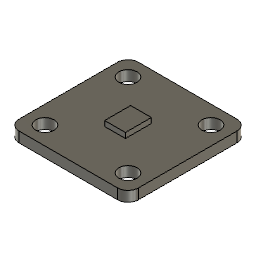
Leg Assembly 2026-01-18 (Autodesk Fusion 360 archive; units mm, degrees)
design "encoderBB"
Autodesk Fusion 360 part; units mm, degrees
sketch "Sketch1" plane through (0, 0, 0) normal (0, 0, 1) x (1, 0, 0)
  line L0 (8, -8) -> (-8, -8)
  line L1 (-8, -8) -> (-8, 8)
  line L2 (-8, 8) -> (8, 8)
  line L3 (8, 8) -> (8, -8)
  line L4 (8, -8) -> (-8, 8) construction
  line L5 (-8, -8) -> (8, 8) construction
  circle A0 centre (-8, 8) radius 1.75
  circle A1 centre (-8, -8) radius 1.75
  circle A2 centre (8, -8) radius 1.75
  circle A3 centre (8, 8) radius 1.75
  line L6 (11.5, -11.5) -> (-11.5, -11.5)
  line L7 (-11.5, -11.5) -> (-11.5, 11.5)
  line L8 (-11.5, 11.5) -> (11.5, 11.5)
  line L9 (11.5, 11.5) -> (11.5, -11.5)
  line L10 (11.5, -11.5) -> (-11.5, 11.5) construction
  line L11 (-11.5, -11.5) -> (11.5, 11.5) construction
  dimension "d1" = 16
  dimension "d2" = 16
  dimension "d3" = 3.5
  dimension "d4" = 3.5
  dimension "d5" = 3.5
  dimension "d6" = 3.5
  dimension "d7" = 23
  dimension "d8" = 23
  constraint horizontal L0
  constraint perpendicular L0 L1
  constraint parallel L0 L2
  constraint parallel L1 L3
  constraint coincident L4 origin
  constraint coincident L5 origin
  constraint coincident L1.end L2.start
  constraint coincident L0.end L1.start
  constraint coincident L0.start L3.end
  constraint coincident L2.end L3.start
  constraint horizontal L6
  constraint perpendicular L6 L7
  constraint parallel L6 L8
  constraint parallel L7 L9
  constraint coincident L10 origin
  constraint coincident L11 origin
  measures "d1" distance of L1.end L2.end
  measures "d2" distance of L0.end L1.end
  measures "d3" diameter of A0
  measures "d4" diameter of A1
  measures "d5" diameter of A2
  measures "d6" diameter of A3
  measures "d7" distance of L7.end L8.end
  measures "d8" distance of L6.end L7.end
extrude "Extrude1" add sketch "Sketch1" along normal blind 2 contours L0 L1 L2 L3 A0 A1 A2 A3 | L6 L7 L8 L9
fillet "Fillet1" radius 2 4 edges at (-11.5, 11.5, 1) (-11.5, -11.5, 1) (11.5, -11.5, 1) (11.5, 11.5, 1)
sketch "Sketch2" plane through (0, 0, 2) normal (0, 0, 1) x (-1, 0, 0)
  arc A0 (-11.5, -9.5) -> (-9.5, -11.5) centre (-9.5, -9.5) ccw
  line L0 (-9.5, -11.5) -> (9.5, -11.5)
  arc A1 (9.5, -11.5) -> (11.5, -9.5) centre (9.5, -9.5) ccw
  line L1 (11.5, -9.5) -> (11.5, 9.5)
  arc A2 (11.5, 9.5) -> (9.5, 11.5) centre (9.5, 9.5) ccw
  line L2 (9.5, 11.5) -> (-9.5, 11.5)
  arc A3 (-9.5, 11.5) -> (-11.5, 9.5) centre (-9.5, 9.5) ccw
  line L3 (-11.5, 9.5) -> (-11.5, -9.5)
  circle A4 centre (-8, -8) radius 1.75
  circle A5 centre (8, 8) radius 1.75
  circle A6 centre (-8, 8) radius 1.75
  circle A7 centre (8, -8) radius 1.75
  line L4 (-2, 2.5) -> (2, 2.5)
  line L5 (2, 2.5) -> (2, -2.5)
  line L6 (2, -2.5) -> (-2, -2.5)
  line L7 (-2, -2.5) -> (-2, 2.5)
  line L8 (-2, 2.5) -> (2, -2.5) construction
  line L9 (2, 2.5) -> (-2, -2.5) construction
  dimension "d13" = 4
  dimension "d14" = 5
  constraint horizontal L4
  constraint perpendicular L4 L5
  constraint parallel L4 L6
  constraint parallel L5 L7
  constraint coincident L8 origin
  constraint coincident L9 origin
  measures "d13" distance of L5.end L6.end
  measures "d14" distance of L4.end L5.end
extrude "Extrude2" add sketch "Sketch2" along normal blind 1 contours L4 L5 L6 L7

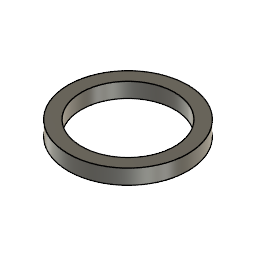
design "25mm id bearing"
Autodesk Fusion 360 part; units mm, degrees
sketch "Sketch1" plane through (0, 0, 0) normal (0, 0, 1) x (1, 0, 0)
  circle A0 centre (0, 0) radius 12.5
  circle A1 centre (0, 0) radius 16
  dimension "d1" = 25
  dimension "d2" = 32
  constraint coincident A0.centre A1.centre
  measures "d1" diameter of A0
  measures "d2" diameter of A1
extrude "Extrude1" add sketch "Sketch1" along normal blind 4

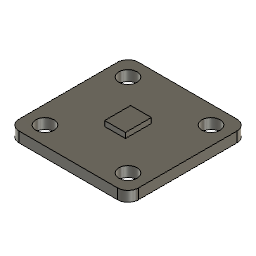
design "encoderBB"
Autodesk Fusion 360 part; units mm, degrees
sketch "Sketch1" plane through (0, 0, 0) normal (0, 0, 1) x (1, 0, 0)
  line L0 (8, -8) -> (-8, -8)
  line L1 (-8, -8) -> (-8, 8)
  line L2 (-8, 8) -> (8, 8)
  line L3 (8, 8) -> (8, -8)
  line L4 (8, -8) -> (-8, 8) construction
  line L5 (-8, -8) -> (8, 8) construction
  circle A0 centre (-8, 8) radius 1.75
  circle A1 centre (-8, -8) radius 1.75
  circle A2 centre (8, -8) radius 1.75
  circle A3 centre (8, 8) radius 1.75
  line L6 (11.5, -11.5) -> (-11.5, -11.5)
  line L7 (-11.5, -11.5) -> (-11.5, 11.5)
  line L8 (-11.5, 11.5) -> (11.5, 11.5)
  line L9 (11.5, 11.5) -> (11.5, -11.5)
  line L10 (11.5, -11.5) -> (-11.5, 11.5) construction
  line L11 (-11.5, -11.5) -> (11.5, 11.5) construction
  dimension "d1" = 16
  dimension "d2" = 16
  dimension "d3" = 3.5
  dimension "d4" = 3.5
  dimension "d5" = 3.5
  dimension "d6" = 3.5
  dimension "d7" = 23
  dimension "d8" = 23
  constraint horizontal L0
  constraint perpendicular L0 L1
  constraint parallel L0 L2
  constraint parallel L1 L3
  constraint coincident L4 origin
  constraint coincident L5 origin
  constraint coincident L1.end L2.start
  constraint coincident L0.end L1.start
  constraint coincident L0.start L3.end
  constraint coincident L2.end L3.start
  constraint horizontal L6
  constraint perpendicular L6 L7
  constraint parallel L6 L8
  constraint parallel L7 L9
  constraint coincident L10 origin
  constraint coincident L11 origin
  measures "d1" distance of L1.end L2.end
  measures "d2" distance of L0.end L1.end
  measures "d3" diameter of A0
  measures "d4" diameter of A1
  measures "d5" diameter of A2
  measures "d6" diameter of A3
  measures "d7" distance of L7.end L8.end
  measures "d8" distance of L6.end L7.end
extrude "Extrude1" add sketch "Sketch1" along normal blind 2 contours L0 L1 L2 L3 A0 A1 A2 A3 | L6 L7 L8 L9
fillet "Fillet1" radius 2 4 edges at (-11.5, 11.5, 1) (-11.5, -11.5, 1) (11.5, -11.5, 1) (11.5, 11.5, 1)
sketch "Sketch2" plane through (0, 0, 2) normal (0, 0, 1) x (-1, 0, 0)
  arc A0 (-11.5, -9.5) -> (-9.5, -11.5) centre (-9.5, -9.5) ccw
  line L0 (-9.5, -11.5) -> (9.5, -11.5)
  arc A1 (9.5, -11.5) -> (11.5, -9.5) centre (9.5, -9.5) ccw
  line L1 (11.5, -9.5) -> (11.5, 9.5)
  arc A2 (11.5, 9.5) -> (9.5, 11.5) centre (9.5, 9.5) ccw
  line L2 (9.5, 11.5) -> (-9.5, 11.5)
  arc A3 (-9.5, 11.5) -> (-11.5, 9.5) centre (-9.5, 9.5) ccw
  line L3 (-11.5, 9.5) -> (-11.5, -9.5)
  circle A4 centre (-8, -8) radius 1.75
  circle A5 centre (8, 8) radius 1.75
  circle A6 centre (-8, 8) radius 1.75
  circle A7 centre (8, -8) radius 1.75
  line L4 (-2, 2.5) -> (2, 2.5)
  line L5 (2, 2.5) -> (2, -2.5)
  line L6 (2, -2.5) -> (-2, -2.5)
  line L7 (-2, -2.5) -> (-2, 2.5)
  line L8 (-2, 2.5) -> (2, -2.5) construction
  line L9 (2, 2.5) -> (-2, -2.5) construction
  dimension "d13" = 4
  dimension "d14" = 5
  constraint horizontal L4
  constraint perpendicular L4 L5
  constraint parallel L4 L6
  constraint parallel L5 L7
  constraint coincident L8 origin
  constraint coincident L9 origin
  measures "d13" distance of L5.end L6.end
  measures "d14" distance of L4.end L5.end
extrude "Extrude2" add sketch "Sketch2" along normal blind 1 contours L4 L5 L6 L7

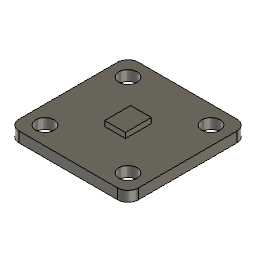
design "encoderBB"
Autodesk Fusion 360 part; units mm, degrees
sketch "Sketch1" plane through (0, 0, 0) normal (0, 0, 1) x (1, 0, 0)
  line L0 (8, -8) -> (-8, -8)
  line L1 (-8, -8) -> (-8, 8)
  line L2 (-8, 8) -> (8, 8)
  line L3 (8, 8) -> (8, -8)
  line L4 (8, -8) -> (-8, 8) construction
  line L5 (-8, -8) -> (8, 8) construction
  circle A0 centre (-8, 8) radius 1.75
  circle A1 centre (-8, -8) radius 1.75
  circle A2 centre (8, -8) radius 1.75
  circle A3 centre (8, 8) radius 1.75
  line L6 (11.5, -11.5) -> (-11.5, -11.5)
  line L7 (-11.5, -11.5) -> (-11.5, 11.5)
  line L8 (-11.5, 11.5) -> (11.5, 11.5)
  line L9 (11.5, 11.5) -> (11.5, -11.5)
  line L10 (11.5, -11.5) -> (-11.5, 11.5) construction
  line L11 (-11.5, -11.5) -> (11.5, 11.5) construction
  dimension "d1" = 16
  dimension "d2" = 16
  dimension "d3" = 3.5
  dimension "d4" = 3.5
  dimension "d5" = 3.5
  dimension "d6" = 3.5
  dimension "d7" = 23
  dimension "d8" = 23
  constraint horizontal L0
  constraint perpendicular L0 L1
  constraint parallel L0 L2
  constraint parallel L1 L3
  constraint coincident L4 origin
  constraint coincident L5 origin
  constraint coincident L1.end L2.start
  constraint coincident L0.end L1.start
  constraint coincident L0.start L3.end
  constraint coincident L2.end L3.start
  constraint horizontal L6
  constraint perpendicular L6 L7
  constraint parallel L6 L8
  constraint parallel L7 L9
  constraint coincident L10 origin
  constraint coincident L11 origin
  measures "d1" distance of L1.end L2.end
  measures "d2" distance of L0.end L1.end
  measures "d3" diameter of A0
  measures "d4" diameter of A1
  measures "d5" diameter of A2
  measures "d6" diameter of A3
  measures "d7" distance of L7.end L8.end
  measures "d8" distance of L6.end L7.end
extrude "Extrude1" add sketch "Sketch1" along normal blind 2 contours L0 L1 L2 L3 A0 A1 A2 A3 | L6 L7 L8 L9
fillet "Fillet1" radius 2 4 edges at (-11.5, 11.5, 1) (-11.5, -11.5, 1) (11.5, -11.5, 1) (11.5, 11.5, 1)
sketch "Sketch2" plane through (0, 0, 2) normal (0, 0, 1) x (-1, 0, 0)
  arc A0 (-11.5, -9.5) -> (-9.5, -11.5) centre (-9.5, -9.5) ccw
  line L0 (-9.5, -11.5) -> (9.5, -11.5)
  arc A1 (9.5, -11.5) -> (11.5, -9.5) centre (9.5, -9.5) ccw
  line L1 (11.5, -9.5) -> (11.5, 9.5)
  arc A2 (11.5, 9.5) -> (9.5, 11.5) centre (9.5, 9.5) ccw
  line L2 (9.5, 11.5) -> (-9.5, 11.5)
  arc A3 (-9.5, 11.5) -> (-11.5, 9.5) centre (-9.5, 9.5) ccw
  line L3 (-11.5, 9.5) -> (-11.5, -9.5)
  circle A4 centre (-8, -8) radius 1.75
  circle A5 centre (8, 8) radius 1.75
  circle A6 centre (-8, 8) radius 1.75
  circle A7 centre (8, -8) radius 1.75
  line L4 (-2, 2.5) -> (2, 2.5)
  line L5 (2, 2.5) -> (2, -2.5)
  line L6 (2, -2.5) -> (-2, -2.5)
  line L7 (-2, -2.5) -> (-2, 2.5)
  line L8 (-2, 2.5) -> (2, -2.5) construction
  line L9 (2, 2.5) -> (-2, -2.5) construction
  dimension "d13" = 4
  dimension "d14" = 5
  constraint horizontal L4
  constraint perpendicular L4 L5
  constraint parallel L4 L6
  constraint parallel L5 L7
  constraint coincident L8 origin
  constraint coincident L9 origin
  measures "d13" distance of L5.end L6.end
  measures "d14" distance of L4.end L5.end
extrude "Extrude2" add sketch "Sketch2" along normal blind 1 contours L4 L5 L6 L7
